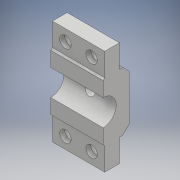
# Autodesk Inventor part: Upper Base Bearing Holder
Saved by Autodesk Inventor 2017 (Build 210142000, 142)
## iProperties
Created: 2018-11-17
Part Number: Upper Base Bearing Holder
Material: Generic
Document SubType Name: Modeling
Designer: Arman Grewal
Density: 1 g/cm^3
Appearance: Default
Author: Arman Grewal
Autodesk Inventor part; units mm, degrees
ref_plane "YZ Plane" through (0, 0, 0) normal (1, 0, 0) x (0, 1, 0)
ref_plane "XZ Plane" through (0, 0, 0) normal (0, 1, 0) x (-1, 0, 0)
ref_plane "XY Plane" through (0, 0, 0) normal (0, 0, 1) x (1, 0, 0)
sketch "Sketch3" plane through (0, 0, 0) normal (0, 1, 0) x (-1, 0, 0)
  line L0 (-8, 16) -> (8, 16)
  line L1 (8, 16) -> (8, -16)
  line L2 (8, -16) -> (-8, -16)
  line L3 (-8, -16) -> (-8, 16)
  line L4 (-8, 16) -> (8, -16) construction
  line L5 (8, 16) -> (-8, -16) construction
  point P0 (0, 0)
  dimension "d7" = 16
  dimension "d8" = 32
  constraints: 12 end point, 2 midpoint, 2 parallel, 1 horizontal, 1 perpendicular
  measures "d7" distance of L1.end L2.end
  measures "d8" distance of L0.end L1.end
extrude "Extrusion1" add sketch "Sketch3" along normal blind 4.5
sketch "Sketch4" plane through (0, 0, 0) normal (0, -1, 0) x (1, 0, 0)
  line L0 (0, 0) -> (0, 9)
  line L1 (0, 9) -> (0, -9)
  line L2 (8, 16) -> (8, -16) projected
  line L3 (-8, -9) -> (8, -9)
  line L4 (8, -9) -> (8, 9)
  line L5 (8, 9) -> (-8, 9)
  line L6 (-8, 9) -> (-8, -9)
  line L7 (-8, -9) -> (8, 9) construction
  line L8 (8, -9) -> (-8, 9) construction
  dimension "d11" = 9
  dimension "d12" = 18
  dimension "d13" = 41.633
  constraints: 16 end point, 2 midpoint, 2 parallel, 2 point on line, 1 horizontal, 1 perpendicular, 1 vertical
  measures "d11" distance of L0.start L0.end
  measures "d12" distance of L0.end L1.end
  measures "d13" angle of L7 L2
extrude "Extrusion2" add sketch "Sketch4" along normal blind 0.5
chamfer "Chamfer1" distance 0.5 angle 45 1 edges at (0, -0.5, 9)
chamfer "Chamfer2" distance 0.5 angle 45 1 edges at (0, -0.5, -9)
sketch "Sketch5" plane through (0, 4.5, 0) normal (0, 1, 0) x (1, 0, 0)
  line L0 (8, -16) -> (8, 16) projected
  line L1 (-8, -9) -> (8, -9)
  line L2 (8, -9) -> (8, 9)
  line L3 (8, 9) -> (-8, 9)
  line L4 (-8, 9) -> (-8, -9)
  line L5 (-8, -9) -> (8, 9) construction
  line L6 (8, -9) -> (-8, 9) construction
  point P0 (0, 0)
  dimension "d22" = 18
  constraints: 12 end point, 2 midpoint, 2 parallel, 1 horizontal, 1 perpendicular, 1 point on line
  measures "d22" distance of L2.end L1.end
extrude "Extrusion3" add sketch "Sketch5" along normal blind 3
chamfer "Chamfer3" distance 2 angle 45 2 edges at (0, 7.5, 9) (0, 7.5, -9)
sketch "Sketch6" plane through (0, 4.5, 0) normal (0, 1, 0) x (1, 0, 0)
  line L0 (-8, -9) -> (-8, -16) construction
  line L1 (-8, -12.5) -> (8, -12.5) construction
  line L2 (8, -9) -> (8, -16) construction
  circle A0 centre (4, -12.5) radius 3 construction
  line L3 (8, -16) -> (-8, -16) construction
  line L4 (0, -16) -> (0, 17.9963) construction
  circle A1 centre (-4, -12.5) radius 3 construction
  line L5 (-8, -8.5) -> (-8, 8.5) construction
  line L6 (-8, 0) -> (8, 0) construction
  line L7 (8, 8.5) -> (8, -8.5) construction
  circle A2 centre (4, 12.5) radius 3 construction
  circle A3 centre (-4, 12.5) radius 3 construction
  circle A4 centre (4, -12.5) radius 3
  circle A5 centre (-4, -12.5) radius 3 construction
  circle A6 centre (-4, -12.5) radius 3
  circle A7 centre (4, 12.5) radius 3 construction
  circle A8 centre (-4, 12.5) radius 3 construction
  circle A9 centre (4, 12.5) radius 3
  circle A10 centre (-4, 12.5) radius 3 construction
  circle A11 centre (-4, 12.5) radius 3
  point P0 (0, 0)
  dimension "d28" = 6
  dimension "d29" = 4
  dimension "d30" = 33.9963
  constraints: 12 centre point, 10 symmetric about line, 6 end point, 5 midpoint, 4 coincident, 1 equal radius, 1 point on line, 1 vertical, 10 other
  measures "d28" diameter of A0
  measures "d29" distance from line of L4 A0.centre
  measures "d30" distance from line of L4.end L3
extrude "Extrusion4" cut sketch "Sketch6" against normal blind 3
sketch "Sketch7" plane through (0, 4.5, 0) normal (0, 1, 0) x (1, 0, 0)
  circle A0 centre (-4, -12.5) radius 3 construction
  line L0 (-7, -12.5) -> (-4, -12.5) construction
  circle A1 centre (4, -12.5) radius 3 construction
  line L1 (-4, -12.5) -> (4, -12.5) construction
  circle A2 centre (4, 12.5) radius 3 construction
  line L2 (4, -12.5) -> (4, 12.5) construction
  circle A3 centre (-4, 12.5) radius 3 construction
  line L3 (4, 12.5) -> (-4, 12.5) construction
  circle A4 centre (-4, -12.5) radius 1.75
  circle A5 centre (4, -12.5) radius 1.75
  circle A6 centre (4, 12.5) radius 1.75
  circle A7 centre (-4, 12.5) radius 1.75
  point P0 (0, 0)
  dimension "d33" = 3.5
  dimension "d34" = 3.5
  dimension "d35" = 3.5
  dimension "d36" = 3.5
  constraints: 8 end point, 4 centre point, 4 coincident, 2 perpendicular, 1 collinear, 1 horizontal, 1 horizontal alignment, 1 other
  measures "d33" diameter of A4
  measures "d34" diameter of A5
  measures "d35" diameter of A6
  measures "d36" diameter of A7
extrude "Extrusion5" cut sketch "Sketch7" against normal blind 5
sketch "Sketch8" plane through (0, 7.5, 0) normal (0, 1, 0) x (1, 0, 0)
  circle A0 centre (0, 0) radius 1.5
  dimension "d39" = 3
  constraints: 1 centre point, 1 coincident
  measures "d39" diameter of A0
extrude "Extrusion6" cut sketch "Sketch8" against normal blind 99
chamfer "Chamfer4" distance 1 angle 45 1 edges at (-1.5, 7.5, 0)
sketch "Sketch9" plane through (8, 0, 16) normal (1, 0, 0) x (0, 0, -1)
  line L0 (17.5, -0.5) -> (14.5, -0.5) projected
  circle A0 centre (16, -0.5) radius 4
  point P0 (16, 0)
  dimension "d45" = 8
  constraints: 1 centre point, 1 midpoint
  measures "d45" diameter of A0
extrude "Extrusion7" cut sketch "Sketch9" against normal blind 99
body "Solid1"
